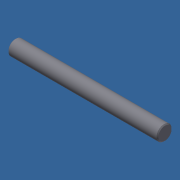
# Autodesk Inventor part: Welle 8x80mm
Saved by Autodesk Inventor 2016 (Build 200138000, 138)
## iProperties
Created: 2015-08-25
Part Number: Welle 8x80mm
Material: Steel
Document SubType Name: Modeling
Designer: 4ndreas
Density: 7.85 g/cm^3
Appearance: Steel
Mass: 31.5195 g
Surface Area: 20.9578 cm^2
Volume: 4.01522 cm^3
CustomPartVersion: 1
Author: 4ndreas
Autodesk Inventor part; units mm, degrees
ref_plane "Startebene" through (0, 0, 0) normal (1, 0, 0) x (0, 1, 0)
ref_plane "XZ Plane" through (0, 0, 0) normal (0, 1, 0) x (-1, 0, 0)
ref_plane "XY Plane" through (0, 0, 0) normal (0, 0, 1) x (1, 0, 0)
sketch "Hauptskizze" plane through (0, 0, 0) normal (0, 0, 1) x (1, 0, 0)
  line L0 (0, 0) -> (80, 0)
  line L1 (0, 0) -> (0, 4)
  line L2 (80, 4) -> (80, 0)
  line L3 (0, 4) -> (80, 4)
  dimension "d3" = 8
  constraints: 8 end point, 2 horizontal, 2 vertical
  measures "d3" diameter of L3 L0
revolve "Umdrehung1" add sketch "Hauptskizze" angle 360 about axis through (0, 0, 0) along (1, 0, 0)
chamfer "Fase4" distance 0.5 angle 45 1 edges at (0, -4, 0) measured on face at (53.3333, 3.9482, -0.6416)
chamfer "Fase2" distance 0.5 angle 45 1 edges at (80, -4, 0) measured on face at (53.5, 3.987, -0.3219)
